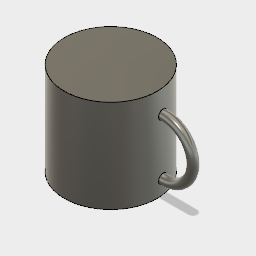
FPROJ_4 (Autodesk Fusion 360 design; units mm, degrees)
Autodesk Fusion 360 part; units mm, degrees
cylinder "圆柱体基本要素1" add diameter 20 height 20 placed x (1, 0, 0) y (0, 0, -1) z (0, 1, 0) at (0, 0, 0) makes body 1
cylinder "圆柱体基本要素2" add diameter 18 height 20 placed x (1, 0, 0) y (0, 0, -1) z (0, 1, 0) at (0, 0, 50) separate body makes body 2
torus "圆环体基本要素1" add centre line diameter 12 section diameter 2 placed x (1, 0, 0) y (0, 0, -1) z (0, 1, 0) at (24.4121, 0, 20.7163) separate body makes body 3
move_body "MoveFace1" bodies 3 to x (1, 0, 0) y (0, 0, -1) z (0, 1, 0) at (-14, -11.7163, -1.2837) on bodies 3
combine "合并1" operation add target body 1 tool bodies 3
move_body "对齐1" bodies 2 to x (1, 0, 0) y (0, 1, 0) z (0, 0, 1) at (0, 0, 0)
move_body "对齐2" bodies 2 to x (1, 0, 0) y (0, 1, 0) z (0, 0, 1) at (0, 0, 0)
move_body "对齐3" bodies 1 to x (1, 0, 0) y (0, 1, 0) z (0, 0, 1) at (0, 0, 50)
move_face "偏移面1" offset -2 1 faces at (-5.1676, 20, 49.6733) on bodies 2
combine "合并2" operation cut target body 1 tool bodies 2
